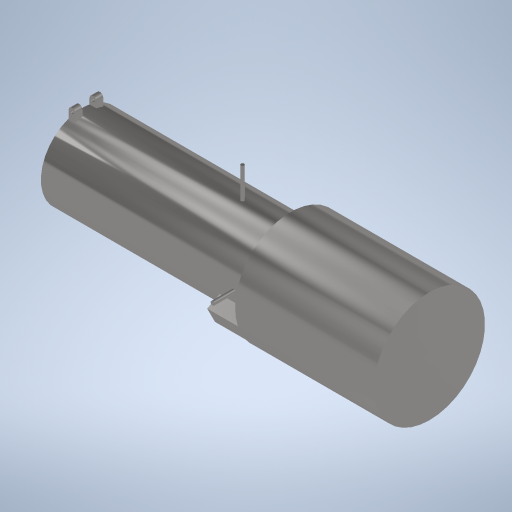
# Autodesk Inventor part: hubble_main_body
Saved by Autodesk Inventor 2024 (Build 280153000, 153)
## iProperties
Created: 2024-04-03
Part Number: hubble_main_body
Material: Stainless Steel AISI 440C, Welded
Document SubType Name: Modeling
Designer: soham
Density: 7.8 g/cm^3
Appearance: Steel - Polished
Author: soham
Autodesk Inventor part; units mm, degrees
sketch "main_body_outline" plane through (0, 0, 0) normal (0, 0, 1) x (1, 0, 0)
  line L0 (0, 0) -> (0, 180)
  line L1 (0, 180) -> (900, 180)
  line L2 (900, 180) -> (900, 240)
  line L3 (900, 240) -> (1500, 240)
  line L4 (1500, 240) -> (1500, 0)
  line L5 (1500, 0) -> (0, 0)
  dimension "d0" = 1500
  dimension "d1" = 900
  dimension "d2" = 240
  dimension "d3" = 180
  constraints: 12 end point, 5 perpendicular, 1 vertical
  measures "d0" distance of L4.end L0.start
  measures "d1" distance of L0.end L1.end
  measures "d2" distance of L3.end L4.end
  measures "d3" distance of L0.start L0.end
revolve "main_body_revolution" add sketch "main_body_outline" angle 360 about axis through (1500, 0, 0) along (-1, 0, 0)
ref_plane "Work Plane1" through (900, 0, 0) normal (1, 0, 0) x (0, 1, 0)
sketch "utility_bay_outline" plane through (900, 0, 0) normal (1, 0, 0) x (0, 1, 0)
  circle A0 centre (0, 0) radius 240 projected
  line L0 (0, 336) -> (0, -336) projected
  circle A1 centre (0, 0) radius 240 projected
  line L1 (-141.0685, -194.1641) -> (-74.1641, -228.2536)
  line L2 (-194.1641, -141.0685) -> (-141.0685, -194.1641)
  line L3 (-228.2536, -74.1641) -> (-194.1641, -141.0685)
  line L4 (-240, 0) -> (-228.2536, -74.1641)
  line L5 (-74.1641, -228.2536) -> (-46.4687, -173.8984)
  circle A2 centre (0, 0) radius 180 projected
  arc A3 (-46.4687, 173.8984) -> (-46.4687, -173.8984) centre (0, 0) ccw
  line L6 (-228.2536, 74.1641) -> (-240, 0)
  line L7 (-194.1641, 141.0685) -> (-228.2536, 74.1641)
  line L8 (-141.0685, 194.1641) -> (-194.1641, 141.0685)
  line L9 (-74.1641, 228.2536) -> (-141.0685, 194.1641)
  line L10 (-46.4687, 173.8984) -> (-74.1641, 228.2536)
  point P0 (-46.4687, 173.8984)
  dimension "d23" = 75.0885
  dimension "d26" = 75.0885
  dimension "d29" = 75.0885
  dimension "d32" = 75.0885
  dimension "d35" = 54.3552
  dimension "d38" = 75.0885
  dimension "d41" = 75.0885
  dimension "d44" = 75.0885
  dimension "d47" = 75.0885
  constraints: 20 end point, 4 point on circle, 2 perpendicular, 1 centre point, 1 coincident, 10 other
  measures "d23" distance of L1.end L1.start
  measures "d26" distance of L1.start L2.start
  measures "d29" distance of L2.start L3.start
  measures "d32" distance of L3.start L4.start
  measures "d35" vertical distance of L1.end L5.end
  measures "d38" distance of L4.start L6.start
  measures "d41" distance of L6.start L7.start
  measures "d44" distance of L7.start L8.start
  measures "d47" distance of L8.start L9.start
extrude "utility_bay_extrude" add sketch "utility_bay_outline" against normal blind 133 contours L10 A2 L5 L1 L2 L3 L4 L6 L7 L8 L9
ref_plane "Work Plane2" through (450, 0, 180) normal (0, 0, 1) x (1, 0, 0)
sketch "solar_panel_joint_outline" plane through (450, 0, 180) normal (0, 0, 1) x (1, 0, 0)
  circle A0 centre (383.5, 0) radius 8.65
  line L0 (450, 240) -> (450, -74.1641) projected
  line L1 (-750, 0) -> (1350, 0) projected
  point P0 (-450, 0)
  dimension "d52" = 66.5
  dimension "d53" = 17.3
  constraints: 1 centre point, 1 point on line
  measures "d52" distance from line of A0.centre L0
  measures "d53" diameter of A0
extrude "solar_panel_joint_extrude" add sketch "solar_panel_joint_outline" along normal blind 91 and the other way blind 0.037
mirror "solar_panel_joint_mirror" about plane through (0, 0, 0) normal (0, 0, 1) of "solar_panel_joint_extrude"
sketch "aperature_hinge_sketch" plane through (0, 0, 0) normal (1, 0, 0) x (0, 1, 0)
  arc A0 (-46.4687, -173.8984) -> (-46.4687, 173.8984) centre (0, 0) ccw projected
  line L0 (177.4824, 30) -> (217.4824, 30)
  line L1 (217.4824, 30) -> (217.4824, 60)
  line L2 (217.4824, 60) -> (169.7056, 60)
  arc A1 (177.4824, 30) -> (169.7056, 60) centre (0, 0) ccw
  line L3 (180, 0) -> (280, 0)
  line L4 (177.4824, -30) -> (217.4824, -30)
  line L5 (217.4824, -30) -> (217.4824, -60)
  line L6 (217.4824, -60) -> (169.7056, -60)
  arc A2 (169.7056, -60) -> (177.4824, -30) centre (0, 0) ccw
  point P0 (0, 0)
  point P1 (169.7056, -60)
  dimension "d61" = 30
  dimension "d63" = 60
  dimension "d74" = 40
  dimension "d86" = 100
  constraints: 14 end point, 7 point on circle, 4 symmetric about line, 2 centre point, 2 horizontal, 2 perpendicular, 1 coincident, 1 other
  measures "d61" distance of L0.end L1.end
  measures "d63" diameter of L0 L3
  measures "d74" distance of L0.start L0.end
  measures "d86" distance of L3.start L3.end
extrude "aperature_hinge_extrude" add sketch "aperature_hinge_sketch" along normal blind 30
ref_plane "Work Plane5" through (30, 169.7056, 60) normal (0, 0, 1) x (1, 0, 0)
sketch "aperature_hinge_slot_sketch" plane through (30, 169.7056, 60) normal (0, 0, 1) x (1, 0, 0)
  circle A0 centre (-15, 31.7768) radius 7.5
  line L0 (-30, 47.7768) -> (0, 47.7768) projected
  line L1 (0, 47.7768) -> (0, 0) projected
  point P0 (-30, -169.7056)
  point P1 (0, 23.8884)
  dimension "d66" = 16
  dimension "d68" = 15
  dimension "d75" = 15
  constraints: 1 centre point, 1 midpoint
  measures "d66" distance from line of L0 A0.centre
  measures "d68" diameter of A0
  measures "d75" distance from line of L1 A0.centre
extrude "aperature_hinge_slot_extrude" cut sketch "aperature_hinge_slot_sketch" against normal through all
fillet "aperature_hinge_top_fillet" radius 15 4 edges at (0, 217.4824, -45) (0, 217.4824, 45) (30, 217.4824, -45) (30, 217.4824, 45)
sketch "telescope_hole" plane through (0, 0, 0) normal (-1, 0, 0) x (0, 0, 1)
  arc A0 (-60, 169.7056) -> (60, 169.7056) centre (0, 0) ccw projected
  circle A1 centre (0, 0) radius 142.5
  dimension "d76" = 285
  constraints: 1 centre point, 1 coincident
  measures "d76" diameter of A1
extrude "telescope_hole_extrude" cut sketch "telescope_hole" against normal blind 450
ref_plane "Work Plane6" through (0, 180, 0) normal (0, 1, 0) x (-1, 0, 0)
sketch "antenna_slot_sketch" plane through (0, 180, 0) normal (0, 1, 0) x (-1, 0, 0)
  line L0 (-900, -240) -> (-900, 240) projected
  line L1 (-900, 180) -> (0, 180) projected
  line L2 (-900, -180) -> (0, -180) projected
  line L3 (-767, -173.8984) -> (-767, 173.8984) projected
  circle A0 centre (-691.9115, 0) radius 7.15
  line L4 (-1080, 0) -> (180, 0) projected
  point P0 (0, 0)
  point P1 (-900, 228.2536)
  point P2 (-900, -228.2536)
  dimension "d80" = 14.3
  dimension "d81" = 75.0885
  constraints: 1 centre point, 1 point on line
  measures "d80" diameter of A0
  measures "d81" distance from line of L3 A0.centre
extrude "antenna_slot_extrude" add sketch "antenna_slot_sketch" along normal blind 133.3333 and the other way blind 0.026
mirror "antenna_slot_mirror" about plane through (0, 0, 0) normal (0, 1, 0) of "antenna_slot_extrude"
equation "\"d0\" = total_length"
equation "\"d1\" = front_end_length"
equation "\"d2\" = rear_radius"
equation "\"d3\" = front_radius"
equation "\"d23\" = bay_width"
equation "\"d26\" = bay_width"
equation "\"d29\" = bay_width"
equation "\"d32\" = bay_width"
equation "\"d38\" = bay_width"
equation "\"d41\" = bay_width"
equation "\"d44\" = bay_width"
equation "\"d47\" = bay_width"
equation "\"d53\" = solar_panel_slot_diameter"
equation "\"d61\" = aperature_hinge_width"
equation "\"d63\" = aperature_hinge_seperation"
equation "\"d74\" = aperature_hinge_height"
equation "\"d64\" = aperature_hinge_width"
equation "\"d66\" = 0.4 * aperature_hinge_height"
equation "\"d68\" = 0.5 * aperature_hinge_width"
equation "\"d75\" = 0.5 * aperature_hinge_width"
equation "\"d77\" = 0.5 * front_end_length"
equation "\"d80\" = antenna_slot_diameter"
equation "\"d81\" = bay_width"
equation "\"total_length\" = 1500"
equation "\"front_end_length\" = 0.6 * total_length"
equation "\"rear_radius\" = 240"
equation "\"front_radius\" = 0.75 * rear_radius"
equation "\"bay_width\" = 0.312869 * rear_radius"
equation "\"solar_panel_slot_diameter\" = 17.3"
equation "\"aperature_hinge_width\" = 30"
equation "\"aperature_hinge_height\" = 40"
equation "\"aperature_hinge_seperation\" = 60"
equation "\"antenna_slot_diameter\" = 14.3"
body "Solid1"
